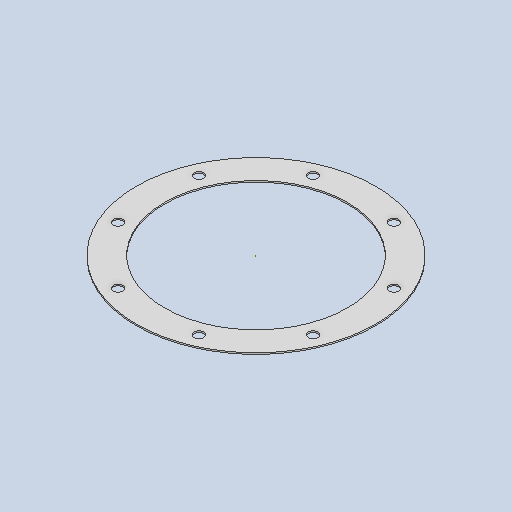
# Autodesk Inventor part: Velcro connection
Saved by Autodesk Inventor 2025.2 (Build 292293000, 293)
## iProperties
Created: 2025-01-13
Part Number: Velcro connection
Material: Generic
Document SubType Name: Modeling
Designer: oskyw
Density: 1 g/cm^3
Appearance: Default
Author: oskyw
Autodesk Inventor part; units mm, degrees
ref_plane "YZ Plane" through (0, 0, 0) normal (1, 0, 0) x (0, 1, 0)
ref_plane "XZ Plane" through (0, 0, 0) normal (0, 1, 0) x (-1, 0, 0)
ref_plane "XY Plane" through (0, 0, 0) normal (0, 0, 1) x (1, 0, 0)
sketch "Sketch1" plane through (0, 0, 0) normal (0, 1, 0) x (-1, 0, 0)
  circle A0 centre (0, 0) radius 65
  circle A1 centre (0, 0) radius 85
  line L0 (0, 0) -> (28.7013, -69.291)
  line L1 (0, 0) -> (0, -65)
  circle A2 centre (28.7013, -69.291) radius 3.5
  circle A3 centre (69.291, -28.7013) radius 3.5
  circle A4 centre (69.291, 28.7013) radius 3.5
  circle A5 centre (28.7013, 69.291) radius 3.5
  circle A6 centre (-28.7013, 69.291) radius 3.5
  circle A7 centre (-69.291, 28.7013) radius 3.5
  circle A8 centre (-69.291, -28.7013) radius 3.5
  circle A9 centre (-28.7013, -69.291) radius 3.5
  dimension "d0" = 130
  dimension "d1" = 170
  dimension "d2" = 22.5
  dimension "d3" = 75
  dimension "d4" = 7
  dimension "d7" = 360
  constraints: 9 centre point, 4 end point, 3 coincident, 1 vertical, 1 vertical alignment, 19 other
  measures "d1" diameter of A1
  measures "d2" angle of L1 L0
  measures "d3" distance of L0.start L0.end
  measures "d4" diameter of A2
extrude "Extrusion1" add sketch "Sketch1" along normal blind 1
equation "\"d3\" = 0.25 * d0 + 0.25 * d1"
body "Solid1"
